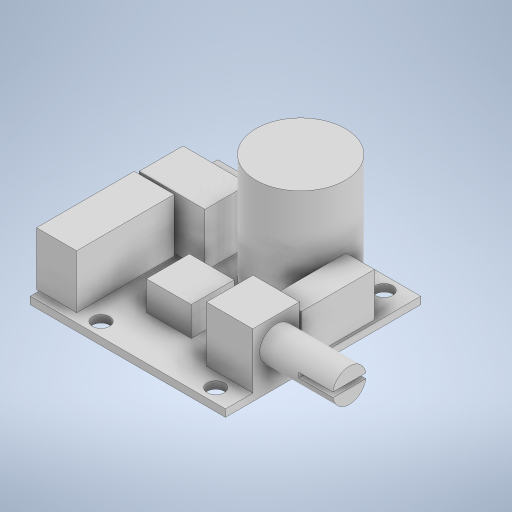
# Autodesk Inventor part: amp
Saved by Autodesk Inventor 2023 (Build 270158000, 158)
## iProperties
Created: 2022-07-14
Part Number: amp
Material: Generic
Document SubType Name: Modeling
Designer: Fuzzyfish
Density: 1 g/cm^3
Appearance: Default
Author: Fuzzyfish
Autodesk Inventor part; units mm, degrees
ref_plane "YZ Plane" through (0, 0, 0) normal (1, 0, 0) x (0, 1, 0)
ref_plane "XZ Plane" through (0, 0, 0) normal (0, 1, 0) x (-1, 0, 0)
ref_plane "XY Plane" through (0, 0, 0) normal (0, 0, 1) x (1, 0, 0)
sketch "Sketch1" plane through (0, 0, 0) normal (0, 1, 0) x (-1, 0, 0)
  line L0 (0, 0) -> (40, 0)
  line L1 (40, 0) -> (40, -40)
  line L2 (40, -40) -> (0, -40)
  line L3 (0, -40) -> (0, 0)
  dimension "d0" = 40
  dimension "d1" = 40
  constraints: 8 end point, 2 parallel, 1 horizontal, 1 perpendicular
  measures "d0" distance of L0.end L1.end
  measures "d1" distance of L1.end L2.end
extrude "Extrusion1" add sketch "Sketch1" along normal blind 1.5
sketch "Sketch2" plane through (0, 1.5, 0) normal (0, 1, 0) x (1, 0, 0)
  circle A0 centre (-4.75, 37.25) radius 1.75
  circle A1 centre (-25.75, 37.25) radius 1.75
  circle A2 centre (-28.25, 2.75) radius 1.75
  circle A3 centre (-4.75, 2.75) radius 1.75
  circle A4 centre (-15.45, 30.85) radius 9.15
  line L0 (-40, 32.4) -> (-29, 32.4)
  line L1 (-29, 32.4) -> (-29, 38.4)
  line L2 (-29, 38.4) -> (-40, 38.4)
  line L3 (-40, 38.4) -> (-40, 32.4)
  line L4 (-40.5, 31.3) -> (-26.5, 31.3)
  line L5 (-26.5, 31.3) -> (-26.5, 22.3)
  line L6 (-26.5, 22.3) -> (-40.5, 22.3)
  line L7 (-40.5, 22.3) -> (-40.5, 31.3)
  line L8 (-40.5, 21.8) -> (-32.3, 21.8)
  line L9 (-32.3, 21.8) -> (-32.3, 1.8)
  line L10 (-32.3, 1.8) -> (-40.5, 1.8)
  line L11 (-40.5, 1.8) -> (-40.5, 21.8)
  line L12 (-9.5, 15.15) -> (0, 15.15)
  line L13 (0, 15.15) -> (0, 5.6)
  line L14 (0, 5.6) -> (-9.5, 5.6)
  line L15 (-9.5, 5.6) -> (-9.5, 15.15)
  line L16 (-6.3, 31) -> (-0.5, 31)
  line L17 (-0.5, 31) -> (-0.5, 16)
  line L18 (-0.5, 16) -> (-6.3, 16)
  line L19 (-6.3, 16) -> (-6.3, 31)
  line L20 (-25.2, 17.8) -> (-16, 17.8)
  line L21 (-16, 17.8) -> (-16, 9)
  line L22 (-16, 9) -> (-25.2, 9)
  line L23 (-25.2, 9) -> (-25.2, 17.8)
  line L24 (-40, 0) -> (0, 0) projected
  line L25 (0, 40) -> (-40, 40) projected
  line L26 (-40, 40) -> (-40, 0) projected
  line L27 (-40, 0) -> (0, 0) projected
  line L28 (0, 0) -> (0, 40) projected
  line L29 (0, 40) -> (-40, 40) projected
  point P0 (-36.4, 1.8)
  point P1 (-40, 31.3)
  point P2 (-40, 22.3)
  dimension "d4" = 3.5
  dimension "d5" = 3.5
  dimension "d6" = 3.5
  dimension "d7" = 3.5
  dimension "d8" = 18.3
  dimension "d9" = 8.2
  dimension "d10" = 20
  dimension "d11" = 8.8
  dimension "d12" = 9.2
  dimension "d13" = 9.55
  dimension "d14" = 9.5
  dimension "d15" = 15
  dimension "d16" = 5.8
  dimension "d17" = 11
  dimension "d18" = 6
  dimension "d21" = 9
  dimension "d22" = 14
  dimension "d23" = 5.6
  dimension "d24" = 4.75
  dimension "d25" = 2.75
  dimension "d26" = 0.5
  dimension "d27" = 9
  dimension "d28" = 9
  dimension "d29" = 6.5
  dimension "d30" = 9.15
  dimension "d31" = 9.15
  dimension "d32" = 2.75
  dimension "d33" = 0.5
  dimension "d34" = 1.8
  dimension "d35" = 1.6
  dimension "d37" = 0.5
  dimension "d38" = 0.5
  dimension "d39" = 11.75
  dimension "d40" = 2.75
  dimension "d41" = 2.75
  dimension "d42" = 4.75
  dimension "d43" = 14.25
  constraints: 48 end point, 12 parallel, 6 horizontal, 6 perpendicular, 5 centre point, 2 point on line, 1 midpoint
  measures "d4" diameter of A0
  measures "d5" diameter of A1
  measures "d6" diameter of A2
  measures "d7" diameter of A3
  measures "d8" diameter of A4
  measures "d9" distance between parallel lines of L11 L9
  measures "d10" distance from line of point (-36.4, 1.8) L8
  measures "d11" distance of L20.end L21.end
  measures "d12" distance of L20.start L20.end
  measures "d13" distance between parallel lines of L12 L14
  measures "d14" distance between parallel lines of L13 L15
  measures "d15" distance of L16.end L17.end
  measures "d16" distance between parallel lines of L17 L19
  measures "d17" distance of L1.end L2.end
  measures "d18" distance of L2.end L0.start
  measures "d21" distance between parallel lines of L6 L4
  measures "d22" distance between parallel lines of L5 L7
  measures "d23" distance between parallel lines of L14 L24
  measures "d24" distance from line of L28 A3.centre
  measures "d25" distance from line of L24 A3.centre
  measures "d26" distance between parallel lines of L28 L17
  measures "d27" distance between parallel lines of L25 L16
  measures "d28" distance between parallel lines of L27 L22
  measures "d29" distance between parallel lines of L15 L21
  measures "d30" distance from line of L25 A4.centre
  measures "d31" distance from line of L19 A4.centre
  measures "d32" distance from line of L24 A2.centre
  measures "d33" distance between parallel lines of L26 L11
  measures "d34" distance between parallel lines of L10 L24
  measures "d35" distance between parallel lines of L25 L2
  measures "d37" distance between parallel lines of L26 L7
  measures "d38" distance between parallel lines of L8 L6
  measures "d39" distance from line of L26 A2.centre
  measures "d40" distance from line of L25 A1.centre
  measures "d41" distance from line of L29 A0.centre
  measures "d42" distance from line of L28 A0.centre
  measures "d43" distance from line of L26 A1.centre
extrude "Extrusion2" add sketch "Sketch2" along normal blind 6 contours L20 L21 L22 L23
extrude "Extrusion3" add sketch "Sketch2" along normal blind 22 contours A4
extrude "Extrusion4" cut sketch "Sketch2" against normal through all contours A0 | A1 | A2 | A3
extrude "Extrusion5" add sketch "Sketch2" along normal blind 11 contours L26 L8 L9 L10 | L10 L11 L8 L26
extrude "Extrusion6" add sketch "Sketch2" along normal blind 11.4 contours L13 L14 L15 L12
sketch "Sketch2 outline for Extrusion7" plane through (0, 1.5, 0) normal (0, 1, 0) x (1, 0, 0)
  line L0 (-6.3, 16) -> (-0.5, 16)
  line L1 (-6.3, 31) -> (-6.3, 16)
  line L2 (-0.5, 31) -> (-6.3, 31)
  line L3 (-0.5, 16) -> (-0.5, 31)
extrude "Extrusion7" add sketch "Sketch2 outline for Extrusion7" along normal blind 9
extrude "Extrusion8" add sketch "Sketch2" along normal blind 11 contours L4 L5 L6 L26
extrude "Extrusion9" add sketch "Sketch2" along normal blind 5 contours L2 L1 L0 L3
sketch "Sketch3" plane through (-40, 0, -40) normal (-1, 0, 0) x (0, 0, 1)
  line L0 (8.7, 12.5) -> (17.7, 12.5) projected
  line L1 (8.7, 1.5) -> (8.7, 12.5) projected
  line L2 (17.7, 1.5) -> (17.7, 12.5) projected
  circle A0 centre (13.2, 7.875) radius 3.125
  point P0 (40, 0)
  dimension "d60" = 6.25
  dimension "d61" = 4.625
  constraints: 1 centre point
  measures "d60" diameter of A0
  measures "d61" distance from line of L0 A0.centre
extrude "Extrusion10" cut sketch "Sketch3" against normal blind 13
sketch "Sketch4" plane through (-40, 0, -40) normal (-1, 0, 0) x (0, 0, 1)
  line L0 (1.6, 1.5) -> (1.6, 6.5) projected
  line L1 (1.6, 6.5) -> (7.6, 6.5) projected
  line L2 (7.6, 1.5) -> (7.6, 6.5) projected
  circle A0 centre (4.6, 4) radius 2.5
  circle A1 centre (4.6, 4) radius 1.5
  point P0 (40, 0)
  dimension "d64" = 5
  dimension "d65" = 1
  dimension "d66" = 6
  dimension "d67" = 3
  constraints: 2 centre point, 1 coincident, 1 tangent
  measures "d64" diameter of A0
  measures "d65" radial gap between concentric circles of A0 A1
  measures "d66" distance between parallel lines of L2 L0
  measures "d67" distance from line of L0 A0.centre
extrude "Extrusion11" add sketch "Sketch4" along normal blind 2.5
sketch "Sketch5" plane through (0, 0, 0) normal (1, 0, 0) x (0, 0, -1)
  circle A0 centre (10.375, 8) radius 3.4
  line L0 (15.15, 1.5) -> (15.15, 12.9) projected
  line L1 (5.6, 12.9) -> (15.15, 12.9) projected
  line L2 (5.6, 1.5) -> (5.6, 12.9) projected
  point P0 (0, 0)
  dimension "d70" = 6.8
  dimension "d71" = 4.9
  dimension "d72" = 4.775
  dimension "d73" = 9.55
  constraints: 1 centre point
  measures "d70" diameter of A0
  measures "d71" distance from line of L1 A0.centre
  measures "d72" distance from line of L0 A0.centre
  measures "d73" distance of L1.start L0.end
extrude "Extrusion12" add sketch "Sketch5" along normal blind 15
sketch "Sketch6" plane through (15, 8, -10.375) normal (1, 0, 0) x (0, 0, -1)
  circle A0 centre (0, 0) radius 3.4
  line L0 (-3.363034, 0.5) -> (3.363034, 0.5)
  line L1 (3.363034, 0.5) -> (3.363034, -0.5)
  line L2 (3.363034, -0.5) -> (-3.363034, -0.5)
  line L3 (-3.363034, -0.5) -> (-3.363034, 0.5)
  line L4 (-3.363034, 0.5) -> (3.363034, -0.5) construction
  line L5 (3.363034, 0.5) -> (-3.363034, -0.5) construction
  point P0 (-3.363034, 0.5)
  point P1 (-3.363034, -0.5)
  point P2 (3.363034, 0.5)
  dimension "d76" = 1
  constraints: 12 end point, 2 midpoint, 2 parallel, 1 horizontal, 1 perpendicular, 2 other
  measures "d76" distance of L0.end L1.end
extrude "Extrusion13" cut sketch "Sketch6" against normal blind 7 contours A0 L1 | L1 L2 L3 L0 | L3 A0
equation "\"d5\" = d4"
equation "\"d6\" = d5"
equation "\"d7\" = d4"
equation "\"d30\" = 0.5 * d8"
equation "\"d31\" = 0.5 * d8"
body "Solid1"
